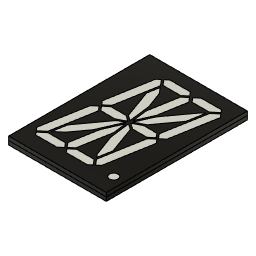
Sixteen Seg Clock v16 (Autodesk Fusion 360 design; units mm, degrees)
Autodesk Fusion 360 part; units mm, degrees
sketch "Sketch1" plane through (0, 0, 0) normal (0, 0, 1) x (1, 0, 0)
  line L0 (0, 0) -> (114.3, 0)
  line L1 (114.3, 0) -> (114.3, 165.1)
  line L2 (114.3, 165.1) -> (0, 165.1)
  line L3 (0, 165.1) -> (0, 0)
  dimension "d1" = 114.3
  dimension "d2" = 165.1
  constraint horizontal L0
  constraint vertical L1
  constraint horizontal L2
  constraint vertical L3
  constraint coincident L0.start L3.end
  measures "d1" distance of L0.start L0.end
  measures "d2" distance of L0.start L2.end
sketch "Sketch2" plane through (0, 0, 0) normal (0, 0, 1) x (1, 0, 0)
  line L0 (114.3, 0) -> (114.3, 165.1)
  line L1 (114.3, 165.1) -> (0, 165.1)
  line L2 (0, 165.1) -> (0, 0)
  line L3 (0, 0) -> (114.3, 0)
  line L4 (37.492, 151.1842) -> (61.492, 151.1842)
  line L5 (38.9364, 141.6842) -> (33.6618, 147.9703)
  line L6 (33.6618, 147.9703) -> (37.492, 151.1842)
  line L7 (68.8731, 146.5879) -> (74.3507, 151.1842)
  line L8 (97.9889, 151.1842) -> (100.5601, 148.12)
  line L9 (100.5601, 148.12) -> (92.8901, 141.6842)
  line L10 (92.8901, 141.6842) -> (72.9878, 141.6842)
  line L11 (72.9878, 141.6842) -> (68.8731, 146.5879)
  line L12 (28.2995, 143.4708) -> (32.1297, 146.6847)
  line L13 (32.1297, 146.6847) -> (37.8239, 139.8986)
  line L14 (37.8239, 139.8986) -> (29.3157, 91.6465)
  line L15 (29.3157, 91.6465) -> (22.7903, 86.171)
  line L16 (22.7903, 86.171) -> (18.9938, 90.6954)
  line L17 (18.9938, 90.6954) -> (28.2995, 143.4708)
  line L18 (39.5021, 137.8986) -> (45.1402, 131.1793)
  line L19 (45.1402, 131.1793) -> (52.154, 111.9092)
  line L20 (37.071, 124.1113) -> (39.5021, 137.8986)
  line L21 (60.9936, 139.9763) -> (66.8049, 144.8525)
  line L22 (66.8049, 144.8525) -> (71.1042, 139.7288)
  line L23 (54.9459, 105.6781) -> (60.9936, 139.9763)
  line L24 (69.6708, 92.564) -> (88.8159, 118.8107)
  line L25 (92.3017, 138.5797) -> (88.5809, 135.4575)
  line L26 (88.5809, 135.4575) -> (66.6852, 105.4398)
  line L27 (83.8242, 89.6617) -> (88.0005, 84.6845)
  line L28 (88.0005, 84.6845) -> (82.0146, 79.6617)
  line L29 (82.0146, 79.6617) -> (65.4413, 79.6617)
  line L30 (68.4109, 89.6617) -> (83.8242, 89.6617)
  line L31 (95.7404, 89.5537) -> (105.1125, 142.705)
  line L32 (105.1125, 142.705) -> (101.8507, 146.5922)
  line L33 (101.8507, 146.5922) -> (94.6852, 140.5797)
  line L34 (94.6852, 140.5797) -> (85.8334, 90.3786)
  line L35 (85.8334, 90.3786) -> (90.333, 85.0163)
  line L36 (90.333, 85.0163) -> (95.7404, 89.5537)
  line L37 (16.8579, 78.5823) -> (7.4838, 25.4194)
  line L38 (7.4838, 25.4194) -> (10.6978, 21.5892)
  line L39 (10.6978, 21.5892) -> (18.0506, 27.759)
  line L40 (18.0506, 27.759) -> (26.9314, 78.1243)
  line L41 (26.9314, 78.1243) -> (22.5437, 83.3533)
  line L42 (22.5437, 83.3533) -> (16.8579, 78.5823)
  line L43 (20.4341, 29.759) -> (23.2883, 45.9454)
  line L44 (23.2883, 45.9454) -> (47.1693, 78.6848)
  line L45 (43, 56) -> (29.2626, 37.1669)
  line L46 (29.2626, 37.1669) -> (20.4341, 29.759)
  line L47 (57.9696, 65.2388) -> (51.316, 27.504)
  line L48 (51.316, 27.504) -> (45.6796, 22.7745)
  line L49 (45.6796, 22.7745) -> (41.2571, 28.045)
  line L50 (41.2571, 28.045) -> (46.8717, 59.8872)
  line L51 (64.5535, 77.8417) -> (76.0315, 46.3064)
  line L52 (76.0315, 46.3064) -> (73.1614, 30.0293)
  line L53 (73.1614, 30.0293) -> (69.899, 33.9173)
  line L54 (69.899, 33.9173) -> (60.7589, 59.0294)
  line L55 (83.7385, 78.4974) -> (74.8396, 28.0293)
  line L56 (74.8396, 28.0293) -> (80.3247, 21.4924)
  line L57 (80.3247, 21.4924) -> (84.1549, 24.7064)
  line L58 (84.1549, 24.7064) -> (93.7381, 79.0557)
  line L59 (93.7381, 79.0557) -> (89.8814, 83.6519)
  line L60 (89.8814, 83.6519) -> (83.7385, 78.4974)
  line L61 (11.9833, 20.0571) -> (19.6533, 26.4929)
  line L62 (19.6533, 26.4929) -> (39.9487, 26.4929)
  line L63 (39.9487, 26.4929) -> (44.3683, 21.2258)
  line L64 (44.3683, 21.2258) -> (39.3237, 16.9929)
  line L65 (39.3237, 16.9929) -> (14.5545, 16.9929)
  line L66 (14.5545, 16.9929) -> (11.9833, 20.0571)
  line L67 (46.9455, 21.2258) -> (53.2225, 26.4929)
  line L68 (53.2225, 26.4929) -> (73.5179, 26.4929)
  line L69 (73.5179, 26.4929) -> (78.7926, 20.2068)
  line L70 (78.7926, 20.2068) -> (74.9623, 16.9929)
  line L71 (74.9623, 16.9929) -> (50.4973, 16.9929)
  line L72 (50.4973, 16.9929) -> (46.9455, 21.2258)
  circle A0 centre (102.5, 20.5) radius 5
  line L73 (61.492, 151.1842) -> (65.3487, 146.5879)
  line L74 (65.3487, 146.5879) -> (59.5047, 141.6842)
  line L75 (33.6618, 147.9703) -> (65.3487, 147.9703) construction
  line L76 (65.3487, 147.9703) -> (65.3487, 146.5879) construction
  line L77 (100.5601, 148.12) -> (68.8731, 148.12) construction
  line L78 (68.8731, 148.12) -> (68.8731, 146.5879) construction
  line L79 (65.3487, 146.5879) -> (68.8731, 146.5879) construction
  line L80 (74.3507, 151.1842) -> (97.9889, 151.1842)
  line L81 (38.9364, 141.6842) -> (59.5047, 141.6842)
  line L82 (52.6791, 151.1842) -> (52.6791, 141.6842) construction
  line L83 (71.1042, 139.7288) -> (65.4359, 107.5819)
  circle A1 centre (56.5571, 84.6617) radius 0.6625 construction
  line L84 (28.2522, 79.6617) -> (24.0758, 84.6389)
  line L85 (24.0758, 84.6389) -> (30.0618, 89.6617)
  line L86 (30.0618, 89.6617) -> (47.6729, 89.6617)
  line L87 (28.2522, 79.6617) -> (44.7032, 79.6617)
  line L88 (37.071, 124.1113) -> (49.0795, 91.1183)
  line L89 (56.0953, 85.5487) -> (57.0189, 83.7747) construction
  line L90 (49.0795, 91.1183) -> (65.4413, 79.6617)
  line L91 (47.6729, 89.6617) -> (64.5535, 77.8417)
  line L92 (55.9835, 83.8425) -> (57.1307, 85.4808) construction
  line L93 (46.8717, 59.8872) -> (66.6852, 105.4398)
  line L94 (65.4359, 107.5819) -> (43, 56)
  line L95 (55.6401, 85.0605) -> (57.4741, 84.2628) construction
  line L96 (52.154, 111.9092) -> (57.9696, 65.2388)
  line L97 (60.7589, 59.0294) -> (54.9459, 105.6781)
  line L98 (57.5494, 84.7853) -> (55.5648, 84.538) construction
  line L99 (44.3683, 21.2258) -> (46.9455, 21.2258) construction
  line L100 (25.8431, 26.4929) -> (25.8431, 16.9929) construction
  line L101 (22.5437, 83.3533) -> (10.6978, 21.5892) construction
  line L102 (89.8814, 83.6519) -> (80.3247, 21.4924) construction
  line L103 (92.3017, 138.5797) -> (88.8159, 118.8107)
  line L104 (44.7032, 79.6617) -> (54.629, 84.791) construction
  line L105 (68.4109, 89.6617) -> (58.4851, 84.5324) construction
  line L106 (47.1693, 78.6848) -> (68.4109, 89.6617)
  line L107 (44.7032, 79.6617) -> (69.6708, 92.564)
  dimension "d3" = 10
  dimension "d7" = 24
  dimension "d16" = 140
  dimension "d17" = 130
  dimension "d18" = 130
  dimension "d19" = 140
  dimension "d20" = 9.5
  dimension "d22" = 5
  dimension "d23" = 6
  dimension "d24" = 4
  dimension "d25" = 5
  dimension "d27" = 130
  dimension "d28" = 140
  dimension "d29" = 140
  dimension "d30" = 130
  dimension "d31" = 130
  dimension "d32" = 140
  dimension "d33" = 130
  dimension "d35" = 2
  dimension "d44" = 2
  dimension "d51" = 130
  dimension "d52" = 140
  dimension "d54" = 2
  dimension "d82" = 10
  dimension "d84" = 2
  dimension "d87" = 145
  dimension "d88" = 145
  dimension "d93" = 2
  dimension "d96" = 7
  dimension "d97" = 2
  dimension "d100" = 9.5
  dimension "d101" = 5
  dimension "d102" = 4
  dimension "d103" = 5
  dimension "d104" = 140
  dimension "d105" = 130
  dimension "d106" = 140
  dimension "d107" = 5
  dimension "d108" = 6
  dimension "d115" = 2
  dimension "d120" = 14
  dimension "d124" = 2
  dimension "d125" = 2
  dimension "d133" = 2
  dimension "d134" = 2
  dimension "d135" = 2
  dimension "d136" = 2
  dimension "d137" = 2
  dimension "d139" = 2
  dimension "d142" = 2
  dimension "d143" = 10
  dimension "d144" = 10
  dimension "d145" = 10
  constraint parallel L1 L4
  constraint horizontal L75
  constraint perpendicular L75 L76
  constraint perpendicular L76 L77
  constraint perpendicular L77 L78
  constraint horizontal L79
  constraint equal L75 L77
  constraint parallel L14 L20
  constraint parallel L11 L22
  constraint perpendicular L15 L16
  constraint perpendicular L35 L36
  constraint perpendicular L59 L60
  constraint perpendicular L27 L28
  constraint perpendicular L7 L11
  constraint perpendicular L73 L74
  constraint perpendicular L12 L13
  constraint perpendicular L21 L22
  constraint perpendicular L32 L33
  constraint perpendicular L38 L39
  constraint perpendicular L61 L66
  constraint perpendicular L63 L64
  constraint perpendicular L67 L72
  constraint perpendicular L69 L70
  constraint perpendicular L8 L9
  constraint perpendicular L5 L6
  constraint perpendicular L48 L49
  constraint perpendicular L41 L42
  constraint collinear L4 L80
  constraint horizontal L81
  constraint collinear L10 L81
  constraint coincident L4 L82.start
  constraint coincident L81 L82.end
  constraint perpendicular L81 L82
  constraint collinear L22 L73
  constraint collinear L7 L21
  constraint collinear L6 L12
  constraint collinear L13 L18
  constraint parallel L14 L17
  constraint parallel L31 L34
  constraint parallel L16 L35
  constraint horizontal L29
  constraint horizontal L30
  constraint parallel L27 L35
  constraint horizontal L86
  constraint horizontal L87
  constraint collinear L29 L87
  constraint midpoint A1.centre L89
  constraint coincident L91 L92.start
  constraint coincident L90 L92.end
  constraint perpendicular L90 L92
  constraint midpoint A1.centre L92
  constraint parallel L90 L91
  constraint parallel L93 L94
  constraint coincident L94 L95.start
  constraint coincident L93 L95.end
  constraint perpendicular L93 L95
  constraint midpoint A1.centre L95
  constraint coincident L97 L98.start
  constraint coincident L96 L98.end
  constraint perpendicular L96 L98
  constraint parallel L96 L97
  constraint midpoint A1.centre L98
  constraint collinear L57 L70
  constraint horizontal L71
  constraint horizontal L68
  constraint collinear L65 L71
  constraint collinear L62 L68
  constraint collinear L47 L83
  constraint parallel L47 L50
  constraint parallel L24 L26
  constraint parallel L19 L88
  constraint collinear L39 L46
  constraint collinear L53 L56
  constraint horizontal L99
  constraint coincident L62 L100.start
  constraint coincident L65 L100.end
  constraint perpendicular L65 L100
  constraint perpendicular L84 L85
  constraint collinear L16 L84
  constraint collinear L42 L85
  constraint collinear L14 L40
  constraint collinear L17 L37
  constraint collinear L34 L55
  constraint parallel L40 L43
  constraint parallel L52 L55
  constraint parallel L48 L67
  constraint equal L62 L68
  constraint equal L101 L102
  constraint collinear L20 L43
  constraint collinear L25 L33
  constraint parallel L9 L33
  constraint collinear L52 L103
  constraint equal L27 L84
  constraint collinear L30 L86
  constraint coincident L91 L104.end
  constraint coincident L90 L105.end
  constraint equal L104 L105
  constraint parallel L105 L107
  constraint parallel L104 L107
  constraint parallel L105 L106
  constraint coincident L89.start L107
  constraint coincident L89.end L106
  constraint collinear L38 L66
  constraint collinear L54 L88
  constraint collinear L19 L51
  constraint collinear L24 L45
  constraint collinear L26 L44
  constraint collinear L23 L50
  measures "d3" diameter of A0
  measures "d7" distance of L4.start L4.end
  measures "d16" angle of L9 L10
  measures "d17" angle of L10 L11
  measures "d18" angle of L5 L81
  measures "d19" angle of L74 L81
  measures "d20" distance of L82.start L82.end
  measures "d22" distance of L4.start L5.end
  measures "d23" distance of L4.end L73.end
  measures "d24" distance of L8.start L8.end
  measures "d25" distance of L12.start L12.end
  measures "d27" angle of L13 L14
  measures "d28" angle of L33 L34
  measures "d29" angle of L21 L23
  measures "d30" angle of L22 L83
  measures "d31" angle of L16 L17
  measures "d32" angle of L37 L42
  measures "d33" angle of L58 L59
  measures "d35" distance of L14 L20
  measures "d44" distance of L5 L13
  measures "d51" angle of L55 L56
  measures "d52" angle of L57 L58
  measures "d54" distance of L28 L60
  measures "d82" distance of L86 L87
  measures "d84" distance of L90 L91
  measures "d87" angle of L86 L91
  measures "d88" angle of L88 L90
  measures "d93" distance of L96 L97
  measures "d96" distance of L34.end L35.end
  measures "d97" distance of L39 L61
  measures "d100" distance of L100.start L100.end
  measures "d101" distance of L37.end L38.end
  measures "d102" distance of L61.start L65.end
  measures "d103" distance of L69.end L70.end
  measures "d104" angle of L61 L62
  measures "d105" angle of L62 L63
  measures "d106" angle of L67 L68
  measures "d107" distance of L56.end L57.end
  measures "d108" distance of L58.end L59.end
  measures "d115" distance of L27 L35
  measures "d120" distance of L18.start L20.start
  measures "d124" distance of L49 L63
  measures "d125" distance of L48 L67
  measures "d133" distance of L34 L103
  measures "d134" distance of L93 L94
  measures "d135" distance of L9 L33
  measures "d136" distance of L15 L85
  measures "d137" distance of L41 L84
  measures "d139" distance of L56 L69
  measures "d142" distance of L106 L107
  measures "d143" distance of L23 L83
  measures "d144" distance of L44 L45
  measures "d145" distance of L51 L54
extrude "Extrude1" add sketch "Sketch2" along normal blind 4.5 contours L0 L1 L2 L3 | L90 L94 L96 L107 | L90 L94 L97 L107 | L90 L94 L107 | L94 L96 L107 | L91 L94 L96 L107 | L90 L97 L107 | L90 L91 L93 L94 L96 L97 L106 L107 | L91 L94 L96 | L90 L93 L97 L107 | L90 L93 L97 | L91 L94 L96 L106 | L91 L96 L106 | L90 L93 L97 L106 | L93 L97 L106 | L91 L93 L106 | L91 L93 L96 L106 | L91 L93 L97 L106 makes body 1
copy_body "Body->Comp1" bodies 1 removing the originals makes body 2 in component "Component"
sketch "Sketch3" plane through (0, 0, 0) normal (0, 0, 1) x (1, 0, 0)
  line L0 (74.9623, 16.9929) -> (50.4973, 16.9929)
  line L1 (50.4973, 16.9929) -> (46.9455, 21.2258)
  line L2 (46.9455, 21.2258) -> (53.2225, 26.4929)
  line L3 (53.2225, 26.4929) -> (73.5179, 26.4929)
  line L4 (73.5179, 26.4929) -> (78.7926, 20.2068)
  line L5 (78.7926, 20.2068) -> (74.9623, 16.9929)
  line L6 (16.8579, 78.5823) -> (22.5437, 83.3533)
  line L7 (22.5437, 83.3533) -> (26.9314, 78.1243)
  line L8 (26.9314, 78.1243) -> (18.0506, 27.759)
  line L9 (18.0506, 27.759) -> (10.6978, 21.5892)
  line L10 (10.6978, 21.5892) -> (7.4838, 25.4194)
  line L11 (7.4838, 25.4194) -> (16.8579, 78.5823)
  circle A0 centre (102.5, 20.5) radius 5
  line L12 (39.3237, 16.9929) -> (14.5545, 16.9929)
  line L13 (14.5545, 16.9929) -> (11.9833, 20.0571)
  line L14 (11.9833, 20.0571) -> (19.6533, 26.4929)
  line L15 (19.6533, 26.4929) -> (39.9487, 26.4929)
  line L16 (39.9487, 26.4929) -> (44.3683, 21.2258)
  line L17 (44.3683, 21.2258) -> (39.3237, 16.9929)
  line L18 (83.7385, 78.4974) -> (89.8814, 83.6519)
  line L19 (89.8814, 83.6519) -> (93.7381, 79.0557)
  line L20 (93.7381, 79.0557) -> (84.1549, 24.7064)
  line L21 (84.1549, 24.7064) -> (80.3247, 21.4924)
  line L22 (80.3247, 21.4924) -> (74.8396, 28.0293)
  line L23 (74.8396, 28.0293) -> (83.7385, 78.4974)
  line L24 (22.7903, 86.171) -> (18.9938, 90.6954)
  line L25 (18.9938, 90.6954) -> (28.2995, 143.4708)
  line L26 (28.2995, 143.4708) -> (32.1297, 146.6847)
  line L27 (32.1297, 146.6847) -> (37.8239, 139.8986)
  line L28 (37.8239, 139.8986) -> (29.3157, 91.6465)
  line L29 (29.3157, 91.6465) -> (22.7903, 86.171)
  line L30 (95.7404, 89.5537) -> (90.333, 85.0163)
  line L31 (90.333, 85.0163) -> (85.8334, 90.3786)
  line L32 (85.8334, 90.3786) -> (94.6852, 140.5797)
  line L33 (94.6852, 140.5797) -> (101.8507, 146.5922)
  line L34 (101.8507, 146.5922) -> (105.1125, 142.705)
  line L35 (105.1125, 142.705) -> (95.7404, 89.5537)
  line L36 (38.9364, 141.6842) -> (33.6618, 147.9703)
  line L37 (33.6618, 147.9703) -> (37.492, 151.1842)
  line L38 (37.492, 151.1842) -> (61.492, 151.1842)
  line L39 (61.492, 151.1842) -> (65.3487, 146.5879)
  line L40 (65.3487, 146.5879) -> (59.5047, 141.6842)
  line L41 (59.5047, 141.6842) -> (38.9364, 141.6842)
  line L42 (68.8731, 146.5879) -> (74.3507, 151.1842)
  line L43 (74.3507, 151.1842) -> (97.9889, 151.1842)
  line L44 (97.9889, 151.1842) -> (100.5601, 148.12)
  line L45 (100.5601, 148.12) -> (92.8901, 141.6842)
  line L46 (92.8901, 141.6842) -> (72.9878, 141.6842)
  line L47 (72.9878, 141.6842) -> (68.8731, 146.5879)
  line L48 (41.2571, 28.045) -> (46.8717, 59.8872)
  line L49 (46.8717, 59.8872) -> (56.0166, 80.9119)
  line L50 (56.0166, 80.9119) -> (57.9696, 65.2388)
  line L51 (57.9696, 65.2388) -> (51.316, 27.504)
  line L52 (51.316, 27.504) -> (45.6796, 22.7745)
  line L53 (45.6796, 22.7745) -> (41.2571, 28.045)
  line L54 (69.899, 33.9173) -> (60.7589, 59.0294)
  line L55 (60.7589, 59.0294) -> (57.8278, 82.5511)
  line L56 (57.8278, 82.5511) -> (64.5535, 77.8417)
  line L57 (64.5535, 77.8417) -> (76.0315, 46.3064)
  line L58 (76.0315, 46.3064) -> (73.1614, 30.0293)
  line L59 (73.1614, 30.0293) -> (69.899, 33.9173)
  line L60 (58.4851, 84.5324) -> (68.4109, 89.6617)
  line L61 (68.4109, 89.6617) -> (83.8242, 89.6617)
  line L62 (83.8242, 89.6617) -> (88.0005, 84.6845)
  line L63 (88.0005, 84.6845) -> (82.0146, 79.6617)
  line L64 (82.0146, 79.6617) -> (65.4413, 79.6617)
  line L65 (65.4413, 79.6617) -> (58.4851, 84.5324)
  line L66 (88.8159, 118.8107) -> (69.6708, 92.564)
  line L67 (69.6708, 92.564) -> (58.5953, 86.8406)
  line L68 (58.5953, 86.8406) -> (66.6852, 105.4398)
  line L69 (66.6852, 105.4398) -> (88.5809, 135.4575)
  line L70 (88.5809, 135.4575) -> (92.3017, 138.5797)
  line L71 (92.3017, 138.5797) -> (88.8159, 118.8107)
  line L72 (71.1042, 139.7288) -> (65.4359, 107.5819)
  line L73 (65.4359, 107.5819) -> (57.0976, 88.4114)
  line L74 (57.0976, 88.4114) -> (54.9459, 105.6781)
  line L75 (54.9459, 105.6781) -> (60.9936, 139.9763)
  line L76 (60.9936, 139.9763) -> (66.8049, 144.8525)
  line L77 (66.8049, 144.8525) -> (71.1042, 139.7288)
  line L78 (49.0795, 91.1183) -> (37.071, 124.1113)
  line L79 (37.071, 124.1113) -> (39.5021, 137.8986)
  line L80 (39.5021, 137.8986) -> (45.1402, 131.1793)
  line L81 (45.1402, 131.1793) -> (52.154, 111.9092)
  line L82 (52.154, 111.9092) -> (55.2863, 86.7722)
  line L83 (55.2863, 86.7722) -> (49.0795, 91.1183)
  line L84 (44.7032, 79.6617) -> (28.2522, 79.6617)
  line L85 (28.2522, 79.6617) -> (24.0758, 84.6389)
  line L86 (24.0758, 84.6389) -> (30.0618, 89.6617)
  line L87 (30.0618, 89.6617) -> (47.6729, 89.6617)
  line L88 (47.6729, 89.6617) -> (54.629, 84.791)
  line L89 (54.629, 84.791) -> (44.7032, 79.6617)
  line L90 (23.2883, 45.9454) -> (47.1693, 78.6848)
  line L91 (47.1693, 78.6848) -> (54.5188, 82.4828)
  line L92 (54.5188, 82.4828) -> (43, 56)
  line L93 (43, 56) -> (29.2626, 37.1669)
  line L94 (29.2626, 37.1669) -> (20.4341, 29.759)
  line L95 (20.4341, 29.759) -> (23.2883, 45.9454)
  line L96 (0, 0) -> (114.3, 0)
  line L97 (114.3, 0) -> (114.3, 165.1)
  line L98 (114.3, 165.1) -> (0, 165.1)
  line L99 (0, 165.1) -> (0, 0)
  line L100 (153.2193, -193.5055) -> (153.2193, -28.4055)
  line L101 (134.6598, -103.9518) -> (129.2523, -108.4892)
  line L102 (38.9193, -28.4055) -> (38.9193, -193.5055)
  line L103 (97.4045, -108.973) -> (107.3302, -103.8438)
  line L104 (62.9952, -108.8666) -> (68.9811, -103.8438)
  line L105 (86.5922, -103.8438) -> (93.5483, -108.7145)
  line L106 (122.7435, -103.8438) -> (126.9198, -108.821)
  line L107 (129.2523, -108.4892) -> (124.7528, -103.1269)
  line L108 (68.2351, -101.859) -> (61.7096, -107.3345)
  line L109 (136.9082, -42.3212) -> (139.4794, -45.3854)
  line L110 (110.0236, -53.7767) -> (104.3552, -85.9235)
  line L111 (72.5811, -45.5352) -> (76.4113, -42.3212)
  line L112 (59.3535, -163.7465) -> (62.2076, -147.56)
  line L113 (67.1715, -113.8438) -> (62.9952, -108.8666)
  line L114 (91.0733, -81.5963) -> (94.2057, -106.7332)
  line L115 (83.2876, -172.2796) -> (78.243, -176.5125)
  line L116 (68.9811, -103.8438) -> (86.5922, -103.8438)
  line L117 (94.2057, -106.7332) -> (87.9988, -102.3871)
  line L118 (62.2076, -147.56) -> (86.0886, -114.8207)
  line L119 (89.4166, -176.5125) -> (85.8648, -172.2796)
  line L120 (80.1764, -165.4604) -> (85.7911, -133.6183)
  line L121 (144.0318, -50.8004) -> (134.6598, -103.9518)
  line L122 (50.9027, -173.4484) -> (58.5726, -167.0125)
  line L123 (58.5726, -167.0125) -> (78.868, -167.0125)
  line L124 (98.424, -51.8212) -> (77.8558, -51.8212)
  line L125 (78.868, -167.0125) -> (83.2876, -172.2796)
  line L126 (90.2353, -166.0015) -> (84.599, -170.731)
  line L127 (55.7772, -114.9231) -> (61.4631, -110.1522)
  line L128 (83.6226, -113.8438) -> (67.1715, -113.8438)
  line L129 (77.8558, -51.8212) -> (72.5811, -45.5352)
  line L130 (53.4738, -176.5125) -> (50.9027, -173.4484)
  line L131 (67.2188, -50.0347) -> (71.049, -46.8208)
  line L132 (119.244, -172.013) -> (113.7589, -165.4762)
  line L133 (99.6782, -134.476) -> (96.7471, -110.9543)
  line L134 (111.9072, -51.8212) -> (107.7924, -46.9175)
  line L135 (107.3302, -103.8438) -> (122.7435, -103.8438)
  line L136 (104.3606, -113.8438) -> (97.4045, -108.973)
  line L137 (105.7243, -48.6529) -> (110.0236, -53.7767)
  line L138 (78.243, -176.5125) -> (53.4738, -176.5125)
  line L139 (61.7096, -107.3345) -> (57.9131, -102.81)
  line L140 (71.049, -46.8208) -> (76.7432, -53.6068)
  line L141 (84.0596, -62.3261) -> (91.0733, -81.5963)
  line L142 (46.4032, -168.0861) -> (55.7772, -114.9231)
  line L143 (100.4113, -42.3212) -> (104.2681, -46.9175)
  line L144 (127.5003, -58.0479) -> (131.2211, -54.9258)
  line L145 (84.599, -170.731) -> (80.1764, -165.4604)
  line L146 (117.7119, -173.2986) -> (113.8817, -176.5125)
  line L147 (49.6171, -171.9163) -> (46.4032, -168.0861)
  line L148 (103.4729, -115.6637) -> (114.9508, -147.1991)
  line L149 (133.6046, -52.9258) -> (140.77, -46.9132)
  line L150 (96.0169, -105.094) -> (93.8653, -87.8273)
  line L151 (56.97, -165.7465) -> (49.6171, -171.9163)
  line L152 (127.7353, -74.6947) -> (108.5902, -100.9414)
  line L153 (113.2701, -42.3212) -> (136.9082, -42.3212)
  line L154 (78.4214, -55.6068) -> (84.0596, -62.3261)
  line L155 (76.7432, -53.6068) -> (68.2351, -101.859)
  line L156 (126.9198, -108.821) -> (120.9339, -113.8438)
  line L157 (124.7528, -103.1269) -> (133.6046, -52.9258)
  line L158 (61.4631, -110.1522) -> (65.8507, -115.3812)
  line L159 (57.9131, -102.81) -> (67.2188, -50.0347)
  line L160 (105.6045, -88.0656) -> (127.5003, -58.0479)
  line L161 (108.8183, -159.5882) -> (99.6782, -134.476)
  line L162 (87.9988, -102.3871) -> (75.9903, -69.3941)
  line L163 (81.9193, -137.5055) -> (68.182, -156.3385)
  line L164 (94.9359, -112.5935) -> (96.889, -128.2666)
  line L165 (75.9903, -69.3941) -> (78.4214, -55.6068)
  line L166 (140.77, -46.9132) -> (144.0318, -50.8004)
  line L167 (153.2193, -28.4055) -> (38.9193, -28.4055)
  line L168 (85.7911, -133.6183) -> (94.9359, -112.5935)
  line L169 (96.889, -128.2666) -> (90.2353, -166.0015)
  line L170 (108.5902, -100.9414) -> (97.5146, -106.6649)
  line L171 (113.8817, -176.5125) -> (89.4166, -176.5125)
  line L172 (76.4113, -42.3212) -> (100.4113, -42.3212)
  line L173 (96.7471, -110.9543) -> (103.4729, -115.6637)
  line L174 (97.5146, -106.6649) -> (105.6045, -88.0656)
  line L175 (113.7589, -165.4762) -> (122.6578, -115.0081)
  line L176 (104.3552, -85.9235) -> (96.0169, -105.094)
  line L177 (38.9193, -193.5055) -> (153.2193, -193.5055)
  circle A1 centre (141.4193, -173.0055) radius 5
  line L178 (122.6578, -115.0081) -> (128.8007, -109.8535)
  line L179 (131.8095, -51.8212) -> (111.9072, -51.8212)
  line L180 (65.8507, -115.3812) -> (56.97, -165.7465)
  line L181 (114.9508, -147.1991) -> (112.0807, -163.4762)
  line L182 (86.0886, -114.8207) -> (93.4382, -111.0227)
  line L183 (107.7924, -46.9175) -> (113.2701, -42.3212)
  line L184 (128.8007, -109.8535) -> (132.6575, -114.4498)
  line L185 (68.182, -156.3385) -> (59.3535, -163.7465)
  line L186 (123.0742, -168.7991) -> (119.244, -172.013)
  line L187 (104.2681, -46.9175) -> (98.424, -51.8212)
  line L188 (92.1418, -167.0125) -> (112.4373, -167.0125)
  line L189 (139.4794, -45.3854) -> (131.8095, -51.8212)
  line L190 (99.9129, -53.5292) -> (105.7243, -48.6529)
  line L191 (120.9339, -113.8438) -> (104.3606, -113.8438)
  line L192 (112.4373, -167.0125) -> (117.7119, -173.2986)
  line L193 (93.8653, -87.8273) -> (99.9129, -53.5292)
  line L194 (132.6575, -114.4498) -> (123.0742, -168.7991)
  line L195 (112.0807, -163.4762) -> (108.8183, -159.5882)
  line L196 (93.5483, -108.7145) -> (83.6226, -113.8438)
  line L197 (93.4382, -111.0227) -> (81.9193, -137.5055)
  line L198 (85.8648, -172.2796) -> (92.1418, -167.0125)
  line L199 (131.2211, -54.9258) -> (127.7353, -74.6947)
  point P0 (38.9193, -193.5055)
extrude "Extrude1'" add sketch "Sketch3" along normal blind 4.5 separate body contours L24 L25 L26 L27 L28 L29 makes body 3 in component "Component'"
extrude "Extrude1''" add sketch "Sketch3" along normal blind 4.5 separate body contours L36 L37 L38 L39 L40 L41 makes body 4 in component "Component''"
extrude "Extrude1'''" add sketch "Sketch3" along normal blind 4.5 separate body contours L42 L43 L44 L45 L46 L47 makes body 5 in component "Component'''"
extrude "Extrude1''''" add sketch "Sketch3" along normal blind 4.5 separate body contours L30 L31 L32 L33 L34 L35 makes body 6 in component "Component''''"
extrude "Extrude1'''''" add sketch "Sketch3" along normal blind 4.5 separate body contours L72 L73 L74 L75 L76 L77 makes body 7 in component "Component'''''"
extrude "Extrude1''''''" add sketch "Sketch3" along normal blind 4.5 separate body contours L78 L79 L80 L81 L82 L83 makes body 8 in component "Component''''''"
extrude "Extrude1'''''''" add sketch "Sketch3" along normal blind 4.5 separate body contours L66 L67 L68 L69 L70 L71 makes body 9 in component "Component'''''''"
extrude "Extrude1''''''''" add sketch "Sketch3" along normal blind 4.5 separate body contours L84 L85 L86 L87 L88 L89 makes body 10 in component "Component''''''''"
extrude "Extrude1'''''''''" add sketch "Sketch3" along normal blind 4.5 separate body contours L60 L61 L62 L63 L64 L65 makes body 11 in component "Component'''''''''"
extrude "Extrude1''''''''''" add sketch "Sketch3" along normal blind 4.5 separate body contours L6 L7 L8 L9 L10 L11 makes body 12 in component "Component''''''''''"
extrude "Extrude1'''''''''''" add sketch "Sketch3" along normal blind 4.5 separate body contours L90 L91 L92 L93 L94 L95 makes body 13 in component "Component'''''''''''"
extrude "Extrude1''''''''''''" add sketch "Sketch3" along normal blind 4.5 separate body contours L48 L49 L50 L51 L52 L53 makes body 14 in component "Component''''''''''''"
extrude "Extrude1'''''''''''''" add sketch "Sketch3" along normal blind 4.5 separate body contours L54 L55 L56 L57 L58 L59 makes body 15 in component "Component'''''''''''''"
extrude "Extrude1''''''''''''''" add sketch "Sketch3" along normal blind 4.5 separate body contours L18 L19 L20 L21 L22 L23 makes body 16 in component "Component''''''''''''''"
extrude "Extrude1'''''''''''''''" add sketch "Sketch3" along normal blind 4.5 separate body contours L12 L13 L14 L15 L16 L17 makes body 17 in component "Component'''''''''''''''"
extrude "Extrude1''''''''''''''''" add sketch "Sketch3" along normal blind 4.5 separate body contours L0 L1 L2 L3 L4 L5 makes body 18 in component "Component''''''''''''''''"
extrude "Extrude1'''''''''''''''''" add sketch "Sketch3" along normal blind 4.5 separate body contours A0 makes body 19 in component "Component'''''''''''''''''"
extrude "Extrude1''''''''''''''''''" add 1 faces at (14.1308, 43.9202, 4.5) along direction (0, 0, 1) blind 4.5 separate body on bodies 12 makes body 20 in component "Component''''''''''''''''''"
extrude "Extrude1'''''''''''''''''''" add 1 faces at (25.5363, 108.6042, 4.5) along direction (0, 0, 1) blind 4.5 separate body on bodies 3 makes body 21 in component "Component'''''''''''''''''''"
extrude "Extrude1''''''''''''''''''''" add 1 faces at (52.8296, 148.0175, 4.5) along direction (0, 0, 1) blind 4.5 separate body on bodies 4 makes body 22 in component "Component''''''''''''''''''''"
extrude "Extrude1'''''''''''''''''''''" add 1 faces at (46.1015, 109.0463, 4.5) along direction (0, 0, 1) blind 4.5 separate body on bodies 8 makes body 23 in component "Component'''''''''''''''''''''"
extrude "Extrude1''''''''''''''''''''''" add 1 faces at (40.8126, 86.3284, 4.5) along direction (0, 0, 1) blind 4.5 separate body on bodies 10 makes body 24 in component "Component''''''''''''''''''''''"
extrude "Extrude1'''''''''''''''''''''''" add 1 faces at (60.4585, 117.7454, 4.5) along direction (0, 0, 1) blind 4.5 separate body on bodies 7 makes body 25 in component "Component'''''''''''''''''''''''"
extrude "Extrude1''''''''''''''''''''''''" add 1 faces at (81.3607, 119.9027, 4.5) along direction (0, 0, 1) blind 4.5 separate body on bodies 9 makes body 26 in component "Component''''''''''''''''''''''''"
extrude "Extrude1'''''''''''''''''''''''''" add 1 faces at (71.9556, 82.995, 4.5) along direction (0, 0, 1) blind 4.5 separate body on bodies 11 makes body 27 in component "Component'''''''''''''''''''''''''"
extrude "Extrude1''''''''''''''''''''''''''" add 1 faces at (88.4099, 148.0175, 4.5) along direction (0, 0, 1) blind 4.5 separate body on bodies 5 makes body 28 in component "Component''''''''''''''''''''''''''"
extrude "Extrude1'''''''''''''''''''''''''''" add 1 faces at (98.5127, 124.2795, 4.5) along direction (0, 0, 1) blind 4.5 separate body on bodies 6 makes body 29 in component "Component'''''''''''''''''''''''''''"
extrude "Extrude1''''''''''''''''''''''''''''" add 1 faces at (87.2105, 60.7531, 4.5) along direction (0, 0, 1) blind 4.5 separate body on bodies 16 makes body 30 in component "Component''''''''''''''''''''''''''''"
extrude "Extrude1'''''''''''''''''''''''''''''" add 1 faces at (67.1146, 61.0592, 4.5) along direction (0, 0, 1) blind 4.5 separate body on bodies 15 makes body 31 in component "Component'''''''''''''''''''''''''''''"
extrude "Extrude1''''''''''''''''''''''''''''''" add 1 faces at (52.0525, 50.8766, 4.5) along direction (0, 0, 1) blind 4.5 separate body on bodies 14 makes body 32 in component "Component''''''''''''''''''''''''''''''"
extrude "Extrude1'''''''''''''''''''''''''''''''" add 1 faces at (37.8192, 60.2101, 4.5) along direction (0, 0, 1) blind 4.5 separate body on bodies 13 makes body 33 in component "Component'''''''''''''''''''''''''''''''"
extrude "Extrude1''''''''''''''''''''''''''''''''" add 1 faces at (24.5105, 20.1596, 4.5) along direction (0, 0, 1) blind 4.5 separate body on bodies 17 makes body 34 in component "Component''''''''''''''''''''''''''''''''"
extrude "Extrude1'''''''''''''''''''''''''''''''''" add 1 faces at (59.5607, 20.1596, 4.5) along direction (0, 0, 1) blind 4.5 separate body on bodies 18 makes body 35 in component "Component'''''''''''''''''''''''''''''''''"
extrude "Extrude1''''''''''''''''''''''''''''''''''" add 1 faces at (102.7156, 19.0699, 4.5) along direction (0, 0, 1) blind 4.5 separate body on bodies 19 makes body 36 in component "Component''''''''''''''''''''''''''''''''''"
component "Component" placed x (1, 0, 0) y (0, 1, 0) z (0, 0, 1) at (0, 0, 0)
component "Component" placed x (1, 0, 0) y (0, 1, 0) z (0, 0, 1) at (0, 0, 4.5)
component "Component'" placed x (1, 0, 0) y (0, 1, 0) z (0, 0, 1) at (0, 0, 0)
component "Component''" placed x (1, 0, 0) y (0, 1, 0) z (0, 0, 1) at (0, 0, 0)
component "Component'''" placed x (1, 0, 0) y (0, 1, 0) z (0, 0, 1) at (0, 0, 0)
component "Component''''" placed x (1, 0, 0) y (0, 1, 0) z (0, 0, 1) at (0, 0, 0)
component "Component'''''" placed x (1, 0, 0) y (0, 1, 0) z (0, 0, 1) at (0, 0, 0)
component "Component''''''" placed x (1, 0, 0) y (0, 1, 0) z (0, 0, 1) at (0, 0, 0)
component "Component'''''''" placed x (1, 0, 0) y (0, 1, 0) z (0, 0, 1) at (0, 0, 0)
component "Component''''''''" placed x (1, 0, 0) y (0, 1, 0) z (0, 0, 1) at (0, 0, 0)
component "Component'''''''''" placed x (1, 0, 0) y (0, 1, 0) z (0, 0, 1) at (0, 0, 0)
component "Component''''''''''" placed x (1, 0, 0) y (0, 1, 0) z (0, 0, 1) at (0, 0, 0)
component "Component'''''''''''" placed x (1, 0, 0) y (0, 1, 0) z (0, 0, 1) at (0, 0, 0)
component "Component''''''''''''" placed x (1, 0, 0) y (0, 1, 0) z (0, 0, 1) at (0, 0, 0)
component "Component'''''''''''''" placed x (1, 0, 0) y (0, 1, 0) z (0, 0, 1) at (0, 0, 0)
component "Component''''''''''''''" placed x (1, 0, 0) y (0, 1, 0) z (0, 0, 1) at (0, 0, 0)
component "Component'''''''''''''''" placed x (1, 0, 0) y (0, 1, 0) z (0, 0, 1) at (0, 0, 0)
component "Component''''''''''''''''" placed x (1, 0, 0) y (0, 1, 0) z (0, 0, 1) at (0, 0, 0)
component "Component'''''''''''''''''" placed x (1, 0, 0) y (0, 1, 0) z (0, 0, 1) at (0, 0, 0)
component "Component''''''''''''''''''" placed x (1, 0, 0) y (0, 1, 0) z (0, 0, 1) at (0, 0, 0)
component "Component'''''''''''''''''''" placed x (1, 0, 0) y (0, 1, 0) z (0, 0, 1) at (0, 0, 0)
component "Component''''''''''''''''''''" placed x (1, 0, 0) y (0, 1, 0) z (0, 0, 1) at (0, 0, 0)
component "Component'''''''''''''''''''''" placed x (1, 0, 0) y (0, 1, 0) z (0, 0, 1) at (0, 0, 0)
component "Component''''''''''''''''''''''" placed x (1, 0, 0) y (0, 1, 0) z (0, 0, 1) at (0, 0, 0)
component "Component'''''''''''''''''''''''" placed x (1, 0, 0) y (0, 1, 0) z (0, 0, 1) at (0, 0, 0)
component "Component''''''''''''''''''''''''" placed x (1, 0, 0) y (0, 1, 0) z (0, 0, 1) at (0, 0, 0)
component "Component'''''''''''''''''''''''''" placed x (1, 0, 0) y (0, 1, 0) z (0, 0, 1) at (0, 0, 0)
component "Component''''''''''''''''''''''''''" placed x (1, 0, 0) y (0, 1, 0) z (0, 0, 1) at (0, 0, 0)
component "Component'''''''''''''''''''''''''''" placed x (1, 0, 0) y (0, 1, 0) z (0, 0, 1) at (0, 0, 0)
component "Component''''''''''''''''''''''''''''" placed x (1, 0, 0) y (0, 1, 0) z (0, 0, 1) at (0, 0, 0)
component "Component'''''''''''''''''''''''''''''" placed x (1, 0, 0) y (0, 1, 0) z (0, 0, 1) at (0, 0, 0)
component "Component''''''''''''''''''''''''''''''" placed x (1, 0, 0) y (0, 1, 0) z (0, 0, 1) at (0, 0, 0)
component "Component'''''''''''''''''''''''''''''''" placed x (1, 0, 0) y (0, 1, 0) z (0, 0, 1) at (0, 0, 0)
component "Component''''''''''''''''''''''''''''''''" placed x (1, 0, 0) y (0, 1, 0) z (0, 0, 1) at (0, 0, 0)
component "Component'''''''''''''''''''''''''''''''''" placed x (1, 0, 0) y (0, 1, 0) z (0, 0, 1) at (0, 0, 0)
component "Component''''''''''''''''''''''''''''''''''" placed x (1, 0, 0) y (0, 1, 0) z (0, 0, 1) at (0, 0, 0)
